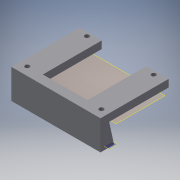
# Autodesk Inventor part: camera_holder
Saved by Autodesk Inventor 2018 (Build 220112000, 112)
## iProperties
Created: 2018-05-16
Part Number: camera_holder
Material: Generic
Document SubType Name: Modeling
Designer: bitbots
Density: 1 g/cm^3
Appearance: Default
Author: bitbots
Autodesk Inventor part; units mm, degrees
ref_plane "YZ Plane" through (0, 0, 0) normal (1, 0, 0) x (0, 1, 0)
ref_plane "XZ Plane" through (0, 0, 0) normal (0, 1, 0) x (-1, 0, 0)
ref_plane "Work Plane1" through (0, 0, 1) normal (0, 0, 1) x (1, 0, 0)
sketch "Sketch2" plane through (0, 0, 1) normal (0, 0, 1) x (1, 0, 0)
  line L0 (-29.9972, 16.3668) -> (29.9972, 16.3668) construction
  line L1 (29.9972, -16.3668) -> (-29.9972, -16.3668) construction
  circle A0 centre (0, 0) radius 8 construction
  line L2 (-18, -2.183) -> (-18, 3.067) construction
  line L3 (17.5, -1.0311) -> (17.5, 1.567) construction
  line L4 (0, 16.3668) -> (0, 17.3668) construction
  line L5 (0, -16.3668) -> (0, -17.3668) construction
  line L6 (0, 17.3668) -> (-30, 17.3668) construction
  line L7 (0, 17.3668) -> (30, 17.3668) construction
  line L8 (-30, 17.3668) -> (30, 17.3668) construction
  line L9 (30, 17.3668) -> (30, -17.3668) construction
  line L10 (30, -17.3668) -> (-30, -17.3668) construction
  line L11 (-30, -17.3668) -> (-30, 17.3668) construction
  line L12 (-30, 17.3668) -> (-15, 17.3668)
  line L13 (-15, 17.3668) -> (-15, -17.3668)
  line L14 (-15, -17.3668) -> (-30, -17.3668)
  line L15 (-30, -17.3668) -> (-30, 17.3668)
  line L16 (30, 17.3668) -> (15, 17.3668)
  line L17 (15, 17.3668) -> (15, -17.3668)
  line L18 (15, -17.3668) -> (30, -17.3668)
  line L19 (30, -17.3668) -> (30, 17.3668)
  point P0 (0, 0)
  dimension "d0" = 1
  dimension "d1" = 1
  dimension "d2" = 30
  dimension "d3" = 30
  dimension "d4" = 15
  dimension "d5" = 15
  constraints: 36 end point, 7 horizontal, 6 parallel, 3 perpendicular, 2 midpoint, 2 point on line, 2 vertical, 4 other
  measures "d0" distance of L4.start L4.end
  measures "d1" distance of L5.start L5.end
  measures "d2" distance of L4.end L6.end
  measures "d3" distance of L4.end L7.end
  measures "d4" distance of L13.end L14.end
  measures "d5" distance of L18.end L17.end
extrude "Extrusion1" add sketch "Sketch2" along normal blind 5
ref_plane "Work Plane2" through (0, -13.2935, -27.0771) normal (0, -0.988012, -0.1543769) x (-1, 0, 0)
sketch "Sketch3" plane through (0, -13.2935, -27.0771) normal (0, -0.988012, -0.1543769) x (-1, 0, 0)
  line L0 (15, -28.3694) -> (30, -28.3694) projected
  line L1 (15, -28.3694) -> (15, -33.3094) projected
  line L2 (30, -33.3094) -> (15, -33.3094) projected
  line L3 (30, -28.3694) -> (30, -33.3094) projected
  line L4 (-15, -28.3694) -> (-30, -28.3694) projected
  line L5 (-30, -28.3694) -> (-30, -33.3094) projected
  line L6 (-15, -33.3094) -> (-30, -33.3094) projected
  line L7 (-15, -28.3694) -> (-15, -33.3094) projected
  line L8 (-24.9964, -11.75) -> (24.9964, -11.75) projected
  line L9 (-30, -33.3094) -> (30, -33.3094)
  line L10 (30, -33.3094) -> (30, -11.3094)
  line L11 (30, -11.3094) -> (-30, -11.3094)
  line L12 (-30, -11.3094) -> (-30, -33.3094)
  point P0 (0, -24.7003)
  dimension "d8" = 60
  dimension "d9" = 22
  constraints: 8 end point, 2 parallel, 1 horizontal, 1 perpendicular
  measures "d8" distance of L11.end L10.end
  measures "d9" distance of L10.end L9.end
extrude "Extrusion2" add sketch "Sketch3" along normal blind 5
sketch "Sketch5" plane through (-30, -17.3668, 1) normal (-1, 0, 0) x (0, 0, 1)
  line L0 (0, 0) -> (0, 34.7337) projected
  line L1 (0, 0) -> (5, 0) projected
  line L2 (5, 34.7337) -> (5, 0) projected
  line L3 (0, 34.7337) -> (5, 34.7337) projected
  line L4 (4.833, -1.0688) -> (-16.9033, 2.3275) projected
  line L5 (-16.9033, 2.3275) -> (-17.6752, -2.6126) projected
  line L6 (4.0611, -6.0089) -> (-17.6752, -2.6126) projected
  line L7 (4.833, -1.0688) -> (4.0611, -6.0089) projected
  line L8 (5, 0) -> (5, -6.1556)
  line L9 (4.0611, -6.0089) -> (-17.6752, -2.6126) projected
  line L10 (5, -6.1556) -> (4.0611, -6.0089)
  line L11 (0, 0) -> (5, 0) projected
  line L12 (0, 0) -> (0, -3.0778)
  line L13 (4.833, -1.0688) -> (4.0611, -6.0089) projected
  line L14 (0, -3.0778) -> (4.0611, -6.0089)
  point P0 (-1, 17.3668)
  constraints: 8 end point, 1 collinear, 1 perpendicular, 1 vertical
extrude "Extrusion3" add sketch "Sketch5" against normal up to surface (60 mm away) contours L1 L8 L10 L7 L4 L12 | L4 L7 L14 L12
sketch "Sketch6" plane through (-30, 17.3668, 1) normal (-1, 0, 0) x (0, 0, 1)
  line L0 (0, -35.0474) -> (0, 0) projected
  line L1 (0, -35.0474) -> (-16.9033, -32.4062) projected
  line L2 (-16.9033, -32.4062) -> (-17.6752, -37.3463) projected
  line L3 (-17.6752, -37.3463) -> (5, -40.8893) projected
  line L4 (5, 0) -> (5, -40.8893) projected
  line L5 (0, 0) -> (5, 0) projected
  line L6 (-16.9033, -32.4062) -> (-24.0532, -32.4062)
  line L7 (-24.0532, -32.4062) -> (-24.0532, -41.4181)
  line L8 (-24.0532, -41.4181) -> (-16.9033, -41.4181)
  line L9 (-16.9033, -41.4181) -> (-16.9033, -32.4062)
  line L10 (-16.9033, -32.4062) -> (-14.9033, -32.4062)
  line L11 (-14.9033, -32.4062) -> (-14.9033, -41.4181)
  line L12 (-14.9033, -41.4181) -> (-16.9033, -41.4181)
  line L13 (-16.9033, -41.4181) -> (-16.9033, -32.4062)
  point P0 (-1, -17.3668)
  dimension "d18" = 2
  constraints: 16 end point, 4 parallel, 2 horizontal, 2 perpendicular
  measures "d18" distance of L11.end L12.end
extrude "Extrusion4" cut sketch "Sketch6" against normal through all contours L11 L3 L9 L1 | L1 L10 L11 | L9 L3 L2 | L2 L3 L9 L8 L7 L6 | L11 L12 L9 L3
sketch "Sketch7" plane through (-30, 17.3668, 1) normal (0, 1, 0) x (1, 0, 0)
  line L0 (0, 0) -> (15, 0) projected
  line L1 (0, 0) -> (0, -5) projected
  line L2 (15, -5) -> (0, -5) projected
  line L3 (15, 0) -> (15, -5) projected
  line L4 (60, 0) -> (45, 0) projected
  line L5 (45, 0) -> (45, -5) projected
  line L6 (60, -5) -> (45, -5) projected
  line L7 (60, 0) -> (60, -5) projected
  point P0 (30, 1)
extrude "Extrusion5" add sketch "Sketch7" along normal blind 5
ref_plane "Work Plane3" through (-30, -20.4125, -11.9033) normal (0, 0, -1) x (-1, 0, 0)
sketch "Sketch8" plane through (-30, -20.4125, -11.9033) normal (0, 0, -1) x (-1, 0, 0)
  line L0 (-7.7, 0) -> (-6, 0) projected
  line L1 (-2.3, 5.0607) -> (-7.7, 5.0607) projected
  circle A0 centre (-5, 2.5303) radius 1.5 projected
  line L2 (-7.7, 0) -> (-6, 0) projected
  line L3 (-57.6, 0) -> (-52.4, 0)
  line L4 (-52.4, 0) -> (-52.4, -6.7313)
  line L5 (-52.4, -6.7313) -> (-57.6, -6.7313)
  line L6 (-57.6, -6.7313) -> (-57.6, 0)
  line L7 (-7.6, 1.0292) -> (-2.4, 1.0292)
  line L8 (-2.4, 1.0292) -> (-2.4, -4.6372)
  line L9 (-2.4, -4.6372) -> (-7.6, -4.6372)
  line L10 (-7.6, -4.6372) -> (-7.6, 1.0292)
  line L11 (-6, 0) -> (-2.3, 0) projected
  line L12 (-2.3, 5.0607) -> (-7.7, 5.0607) projected
  line L13 (-6, 0) -> (-2.3, 0) projected
  circle A1 centre (-5, 2.5303) radius 1.5 projected
  line L14 (-7.7, 5.0607) -> (-7.7, 0) projected
  line L15 (-2.3, 0) -> (-2.3, 5.0607) projected
  line L16 (-7.7, 5.0607) -> (-7.7, 0) projected
  line L17 (-2.3, 0) -> (-2.3, 5.0607) projected
  point P0 (-30, 20.4125)
  point P1 (-7.2835, 0)
  point P2 (-2.4, 0)
  point P3 (-7.2835, 0.8465)
  point P4 (-7.6, 1.0292)
  point P5 (-7.6, 4.0314)
  point P6 (-5.8173, 5.0607)
  point P7 (-4.1827, 5.0607)
  point P8 (-2.4, 4.0314)
  constraints: 16 end point, 4 parallel, 2 horizontal, 2 perpendicular
extrude "Extrusion6" [suppressed]
sketch "Sketch9" plane through (-30, -20.4125, -13.9033) normal (0, 0, -1) x (-1, 0, 0)
  circle A0 centre (-55, 2.5303) radius 1.5 projected
  circle A1 centre (-5, 2.5303) radius 1.5 projected
  point P0 (-30, 20.4125)
extrude "Extrusion7" cut sketch "Sketch9" against normal blind 8
sketch "Sketch10" plane through (0, 0, 1) normal (0, 0, -1) x (-1, 0, 0)
  line L0 (15, 22.3649) -> (15, 22.3668) projected
  line L1 (30, 22.3668) -> (30, 22.3649) projected
  line L2 (30, 22.3668) -> (15, 22.3668) projected
  line L3 (-30, 22.3649) -> (-30, 22.3668) projected
  line L4 (-15, 22.3668) -> (-15, 22.3649) projected
  line L5 (-15, 22.3668) -> (-30, 22.3668) projected
  line L6 (-15, 22.3668) -> (-30, 22.3668) projected
  line L7 (-30, 22.3668) -> (-30, 19.8668)
  line L8 (-30, 22.3668) -> (-30, -17.6805) projected
  line L9 (-30, 19.8668) -> (-22.5, 19.8668)
  line L10 (30, 22.3668) -> (30, 19.8668)
  line L11 (30, -17.6805) -> (30, 22.3668) projected
  line L12 (30, 19.8668) -> (22.5, 19.8668)
  circle A0 centre (-22.5, 19.8668) radius 1.5
  circle A1 centre (22.5, 19.8668) radius 1.5
  line L13 (15, 22.3649) -> (30, 22.3649) projected
  line L14 (-30, 22.3649) -> (-15, 22.3649) projected
  point P0 (0, 0)
  point P1 (30, 17.3668)
  point P2 (-30, 17.3668)
  dimension "d24" = 2.5
  dimension "d25" = 7.5
  dimension "d26" = 2.5
  dimension "d27" = 7.5
  dimension "d28" = 3
  dimension "d29" = 3
  constraints: 8 end point, 2 centre point, 2 coincident, 2 perpendicular, 2 point on line
  measures "d24" distance of L3.end L7.end
  measures "d25" distance of L7.end L9.end
  measures "d26" distance of L1.start L10.end
  measures "d27" distance of L10.end L12.end
  measures "d28" diameter of A0
  measures "d29" diameter of A1
extrude "Extrusion8" cut sketch "Sketch10" against normal through all
sketch "Sketch11" plane through (-30, -20.4125, -13.9033) normal (0, 0, -1) x (-1, 0, 0)
  circle A0 centre (-55, 2.5303) radius 1.5 projected
  circle A1 centre (-5, 2.5303) radius 1.5 projected
  point P0 (-30, 20.4125)
extrude "Extrusion9" cut sketch "Sketch11" against normal through all
sketch "Sketch12" plane through (-30, -20.4125, -13.9033) normal (-1, 0, 0) x (0, 0, 1)
  line L0 (0, 5.0607) -> (0, 0) projected
  line L1 (0, 0) -> (19.9033, -3.1099) projected
  line L2 (19.9033, -3.1099) -> (19.9033, 42.7794) projected
  line L3 (14.9033, 42.7794) -> (19.9033, 42.7794) projected
  line L4 (14.9033, 2.732) -> (14.9033, 42.7794) projected
  line L5 (14.9033, 2.732) -> (0, 5.0607) projected
  line L6 (0, 5.0607) -> (0, 6.0607)
  line L7 (6.5941, 4.0303) -> (14.9033, 2.732) projected
  line L8 (0, 6.0607) -> (14.9033, 2.732)
  point P0 (13.9033, 20.4125)
  dimension "d34" = 1
  constraints: 4 end point, 1 vertical
  measures "d34" distance of L0.start L6.end
extrude "Extrusion10" add sketch "Sketch12" against normal up to surface (60 mm away) contours L6 L8 L5
sketch "Sketch13" plane through (-30, -23.5224, 6) normal (-1, 0, 0) x (0, 0, 1)
  line L0 (-19.9033, 4.1402) -> (0, 4.1402) projected
  line L1 (-19.9033, 7.1402) -> (0, 7.1402) projected
  line L2 (-19.9033, 9.1706) -> (-19.9033, 3.1099) construction
  line L3 (-19.9033, 3.1099) -> (0, 0) construction
  line L4 (0, 0) -> (0, 45.8893) construction
  line L5 (-5, 45.8893) -> (0, 45.8893) projected
  line L6 (-5, 5.8419) -> (-5, 45.8893) projected
  line L7 (-5, 5.8419) -> (-19.9033, 9.1706) projected
  line L8 (-19.9033, 3.1099) -> (0, 3.1099)
  line L9 (0, 3.1099) -> (0, 0)
  line L10 (0, 0) -> (-19.9033, 0)
  line L11 (-19.9033, 0) -> (-19.9033, 3.1099)
  point P0 (-6, 23.5224)
  constraints: 8 end point, 2 parallel, 1 horizontal, 1 perpendicular
extrude "Extrusion11" add sketch "Sketch13" against normal up to surface (60 mm away) contours L8 L9 L10 L11
fillet "Fillet1" radius 1 14 edges at (0, -23.5224, 6) (-22.5, 22.3668, 6) (22.5, 22.3668, 6) (-30, -0.5778, 6) (-15, 2.5, 6) (0, -17.3668, 6) (15, 2.5, 6) (30, -0.5778, 6) (-30, -23.5224, -3.9516) (30, -23.5224, -3.9516) (-30, 22.3668, 3.5) (-15, 22.3668, 3.5) (15, 22.3668, 3.5) (30, 22.3668, 3.5)
sketch "Sketch14" plane through (30, -14.3519, -13.9033) normal (0, 0, -1) x (-1, 0, 0)
  circle A0 centre (5, -3.5303) radius 1.5 projected
  circle A1 centre (55, -3.5303) radius 1.5 projected
  line L0 (60, -8.1706) -> (60, 0) projected
  line L1 (60, 0) -> (0, 0) projected
  line L2 (0, 0) -> (0, -8.1706) projected
  line L3 (59, -9.1706) -> (1, -9.1706) projected
  arc A2 (59, -9.1706) -> (60, -8.1706) centre (59, -8.1706) ccw projected
  arc A3 (0, -8.1706) -> (1, -9.1706) centre (1, -8.1706) ccw projected
  point P0 (30, 14.3519)
extrude "Extrusion12" cut sketch "Sketch14" against normal blind 8
sketch "Sketch15" plane through (-30, -17.6805, 1) normal (-1, 0, 0) x (0, 0, 1)
  line L0 (-6.9033, 1.5418) -> (-6.9033, -4.8419) projected
  line L1 (4, 39.0474) -> (4, -4.8419) projected
  line L2 (0, 0) -> (0, 39.0474) projected
  line L3 (0, 0) -> (-6.9033, 1.5418) projected
  line L4 (4, -5.8419) -> (-6.9033, -5.8419) projected
  line L5 (-6.9033, -5.8419) -> (-43.1083, -5.8419)
  line L6 (-43.1083, -5.8419) -> (-43.1083, 9.6282)
  line L7 (-43.1083, 9.6282) -> (-6.9033, 9.6282)
  line L8 (-6.9033, 9.6282) -> (-6.9033, -5.8419)
  line L9 (4, -4.8419) -> (-6.9033, -4.8419) projected
  line L10 (0, 39.0474) -> (4, 39.0474) projected
  point P0 (-1, 17.6805)
  constraints: 8 end point, 2 parallel, 1 horizontal, 1 perpendicular
extrude "Extrusion13" cut sketch "Sketch15" against normal through all contours L0 L8 L5 L6 L7
body "Solid1"
